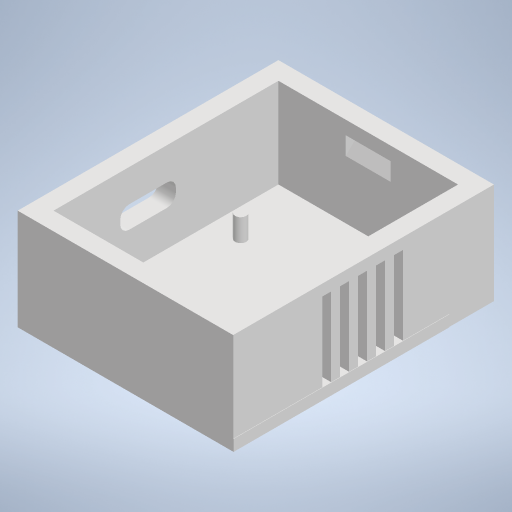
# Autodesk Inventor part: Unterseite
Saved by Autodesk Inventor 2024 (Build 280153000, 153)
## iProperties
Created: 2025-04-30
Part Number: Unterseite
Material: Generisch
Document SubType Name: Modeling
Designer: tobia
Density: 1 g/cm^3
Appearance: Vorgabe
Author: tobia
Autodesk Inventor part; units mm, degrees
ref_plane "YZ Plane" through (0, 0, 0) normal (1, 0, 0) x (0, 1, 0)
ref_plane "XZ Plane" through (0, 0, 0) normal (0, 1, 0) x (-1, 0, 0)
ref_plane "XY Plane" through (0, 0, 0) normal (0, 0, 1) x (1, 0, 0)
sketch "Skizze2" plane through (0, 0, 0) normal (0, 0, 1) x (1, 0, 0)
  line L0 (-24.05, 24.05) -> (24.05, 24.05)
  line L1 (24.05, 24.05) -> (24.05, -24.05)
  line L2 (24.05, -24.05) -> (-24.05, -24.05)
  line L3 (-24.05, -24.05) -> (-24.05, 24.05)
  line L4 (-24.05, 24.05) -> (24.05, -24.05) construction
  line L5 (24.05, 24.05) -> (-24.05, -24.05) construction
  line L6 (24.05, 24.05) -> (20.05, 24.05)
  line L7 (20.05, 24.05) -> (20.05, -24.05)
  line L8 (20.05, -24.05) -> (24.05, -24.05)
  line L9 (24.05, -24.05) -> (24.05, 24.05)
  line L10 (20.05, 24.05) -> (-24.05, 24.05)
  line L11 (-24.05, 24.05) -> (-24.05, 20.05)
  line L12 (-24.05, 20.05) -> (20.05, 20.05)
  line L13 (20.05, 20.05) -> (20.05, 24.05)
  line L14 (-24.05, 20.05) -> (-20.05, 20.05)
  line L15 (-20.05, 20.05) -> (-20.05, -24.05)
  line L16 (-20.05, -24.05) -> (-24.05, -24.05)
  line L17 (-24.05, -24.05) -> (-24.05, 20.05)
  line L18 (-20.05, -24.05) -> (20.05, -24.05)
  line L19 (20.05, -24.05) -> (20.05, -20.05)
  line L20 (20.05, -20.05) -> (-20.05, -20.05)
  line L21 (-20.05, -20.05) -> (-20.05, -24.05)
  point P0 (0, 0)
  dimension "d6" = 48.1
  dimension "d7" = 48.1
  dimension "d8" = 4
  dimension "d9" = 4
  dimension "d10" = 4
  dimension "d11" = 4
  constraints: 44 end point, 10 parallel, 5 horizontal, 5 perpendicular, 4 point on line, 2 midpoint
  measures "d6" distance of L1.end L2.end
  measures "d7" distance of L0.end L1.end
  measures "d8" distance of L8.end L7.end
  measures "d9" distance of L11.end L10.end
  measures "d10" distance of L15.end L16.end
  measures "d11" distance of L19.end L18.end
extrude "Extrusion1" add sketch "Skizze2" against normal blind 2.5
sketch "Skizze3" plane through (0, 0, 0) normal (0, 0, 1) x (1, 0, 0)
  line L0 (-24.05, -24.05) -> (-24.05, 24.05) projected
  line L1 (-24.05, 24.05) -> (-20.05, 24.05)
  line L2 (-20.05, 24.05) -> (-20.05, -24.05)
  line L3 (-20.05, -24.05) -> (-24.05, -24.05)
  line L4 (-24.05, -24.05) -> (-24.05, 24.05)
  line L5 (24.05, 24.05) -> (24.05, -24.05) projected
  line L6 (24.05, 24.05) -> (20.05, 24.05)
  line L7 (20.05, 24.05) -> (20.05, -24.05)
  line L8 (20.05, -24.05) -> (24.05, -24.05)
  line L9 (24.05, -24.05) -> (24.05, 24.05)
  line L10 (20.05, -24.05) -> (-20.05, -24.05)
  line L11 (-20.05, -24.05) -> (-20.05, -20.05)
  line L12 (-20.05, -20.05) -> (20.05, -20.05)
  line L13 (20.05, -20.05) -> (20.05, -24.05)
  line L14 (-20.05, 24.05) -> (20.05, 24.05)
  line L15 (20.05, 24.05) -> (20.05, 20.05)
  line L16 (20.05, 20.05) -> (-20.05, 20.05)
  line L17 (-20.05, 20.05) -> (-20.05, 24.05)
  circle A0 centre (1.0405, -13.9467) radius 1.25
  circle A1 centre (14.1846, 15.3896) radius 1.25
  circle A2 centre (-13.8014, 15.3896) radius 1.25
  point P0 (0, 0)
  dimension "d14" = 4
  dimension "d15" = 4
  dimension "d16" = 4
  dimension "d17" = 4
  dimension "d18" = 2.5
  dimension "d19" = 2.5
  dimension "d20" = 2.5
  constraints: 32 end point, 8 parallel, 4 horizontal, 4 perpendicular, 3 centre point, 3 point on line
  measures "d14" distance of L2.end L3.end
  measures "d15" distance of L8.end L7.end
  measures "d16" distance of L10.end L11.end
  measures "d17" distance of L14.end L15.end
  measures "d18" diameter of A0
  measures "d19" diameter of A1
  measures "d20" diameter of A2
extrude "Extrusion2" add sketch "Skizze3" along normal blind 2.5 contours A0 | A1 | A2
sketch "Skizze4" plane through (-13.8014, 15.3896, 2.5) normal (0, 0, 1) x (1, 0, 0)
  circle A0 centre (27.986, 0) radius 1.25 projected
  circle A1 centre (27.986, 0) radius 1.25
  circle A2 centre (0, 0) radius 1.25 projected
  circle A3 centre (0, 0) radius 1.25
  circle A4 centre (14.8419, -29.3364) radius 1.25 projected
  circle A5 centre (14.8419, -29.3364) radius 1.25
  point P0 (13.8014, -15.3896)
  constraints: 3 centre point, 3 coincident
extrude "Extrusion3" add sketch "Skizze4" along normal blind 2.5
sketch "Skizze5" plane through (-24.05, 24.05, 0) normal (0, 1, 0) x (1, 0, 0)
  line L0 (48.1, 2.5) -> (0, 2.5) projected
  line L1 (48.0134, 0) -> (0, 0)
  line L2 (0, 0) -> (0, 2.5)
  line L3 (0, 2.5) -> (48.0134, 2.5)
  line L4 (48.0134, 2.5) -> (48.0134, 0)
  point P0 (24.05, 0)
  constraints: 8 end point, 2 parallel, 1 horizontal, 1 perpendicular
extrude "Extrusion4" add sketch "Skizze5" along normal blind 10
sketch "Skizze6" plane through (0, 0, 0) normal (0, 0, 1) x (1, 0, 0)
  line L0 (24.05, -24.05) -> (-24.05, -24.05) projected
  line L1 (23.9634, 34.05) -> (-24.05, 34.05) projected
  line L2 (-24.05, -24.05) -> (-20.05, -24.05)
  line L3 (-20.05, -24.05) -> (-20.05, 34.05)
  line L4 (-20.05, 34.05) -> (-24.05, 34.05)
  line L5 (-24.05, 34.05) -> (-24.05, -24.05)
  line L6 (23.9634, 24.05) -> (23.9634, 34.05) projected
  line L7 (-20.05, 34.05) -> (23.9634, 34.05)
  line L8 (23.9634, 34.05) -> (23.9634, 30.05)
  line L9 (23.9634, 30.05) -> (-20.05, 30.05)
  line L10 (-20.05, 30.05) -> (-20.05, 34.05)
  line L11 (23.9634, 30.05) -> (19.9634, 30.05)
  line L12 (19.9634, 30.05) -> (19.9634, -24.05)
  line L13 (19.9634, -24.05) -> (23.9634, -24.05)
  line L14 (23.9634, -24.05) -> (23.9634, 30.05)
  line L15 (19.9634, -24.05) -> (-20.05, -24.05)
  line L16 (-20.05, -24.05) -> (-20.05, -20.05)
  line L17 (-20.05, -20.05) -> (19.9634, -20.05)
  line L18 (19.9634, -20.05) -> (19.9634, -24.05)
  point P0 (0, 0)
  point P1 (-20.05, 30.05)
  dimension "d27" = 4
  dimension "d28" = 4
  dimension "d29" = 4
  dimension "d30" = 4
  constraints: 32 end point, 8 parallel, 4 horizontal, 4 perpendicular, 4 point on line
  measures "d27" distance of L4.end L3.end
  measures "d28" distance of L7.end L8.end
  measures "d29" distance of L13.end L12.end
  measures "d30" distance of L15.end L16.end
extrude "Extrusion5" add sketch "Skizze6" along normal blind 20 contours L0 L12 L9 L6 L14 | L0 L3 L17 L12 | L0 L5 L1 L3 | L9 L3 L1 L6
sketch "Skizze8" plane through (-20.05, -20.05, 0) normal (1, 0, 0) x (0, 0, -1)
  line L0 (-12.8089, 14.8489) -> (-7.8985, 14.8489)
  line L1 (-7.8985, 14.8489) -> (-7.8985, 27.2593)
  line L2 (-7.8985, 27.2593) -> (-12.8089, 27.2593)
  line L3 (-12.8089, 27.2593) -> (-12.8089, 14.8489)
  line L4 (-12.8089, 14.8489) -> (-7.8985, 27.2593) construction
  line L5 (-7.8985, 14.8489) -> (-12.8089, 27.2593) construction
  point P0 (0, 20.05)
  point P1 (-10.3537, 21.0541)
  constraints: 12 end point, 2 midpoint, 2 parallel, 1 horizontal, 1 perpendicular
extrude "Extrusion6" cut sketch "Skizze8" against normal blind 20
fillet "Rundung1" radius 2 4 edges at (-22.05, -5.2011, 12.8089) (-22.05, -5.2011, 7.8985) (-22.05, 7.2093, 12.8089) (-22.05, 7.2093, 7.8985)
sketch "Skizze9" plane through (23.9634, 24.05, 0) normal (1, 0, 0) x (0, 0, -1)
  line L0 (2.5, 10) -> (-20, 10) projected
  line L1 (-20, -48.1) -> (-17.5, -48.1)
  line L2 (-17.5, -48.1) -> (-17.5, 10)
  line L3 (-17.5, 10) -> (-20, 10)
  line L4 (-20, 10) -> (-20, -48.1)
  line L5 (0, -48.1) -> (0, 0) projected
  line L6 (0, -12.2697) -> (-17.5, -12.2697)
  line L7 (-17.5, -12.2697) -> (0, -12.2697)
  line L8 (0, -12.2697) -> (0, -14.2697)
  line L9 (0, -14.2697) -> (-17.5, -14.2697)
  line L10 (-17.5, -14.2697) -> (-17.5, -12.2697)
  line L11 (0, -14.2697) -> (-17.5, -14.2697)
  line L12 (-17.5, -14.2697) -> (-17.5, -16.2697)
  line L13 (-17.5, -16.2697) -> (0, -16.2697)
  line L14 (0, -16.2697) -> (0, -14.2697)
  line L15 (-17.5, -16.2697) -> (0, -16.2697)
  line L16 (0, -16.2697) -> (0, -18.2697)
  line L17 (0, -18.2697) -> (-17.5, -18.2697)
  line L18 (-17.5, -18.2697) -> (-17.5, -16.2697)
  line L19 (0, -18.2697) -> (-17.5, -18.2697)
  line L20 (-17.5, -18.2697) -> (-17.5, -20.2697)
  line L21 (-17.5, -20.2697) -> (0, -20.2697)
  line L22 (0, -20.2697) -> (0, -18.2697)
  line L23 (-17.5, -20.2697) -> (0, -20.2697)
  line L24 (0, -20.2697) -> (0, -22.2697)
  line L25 (0, -22.2697) -> (-17.5, -22.2697)
  line L26 (-17.5, -22.2697) -> (-17.5, -20.2697)
  line L27 (0, -22.2697) -> (-17.5, -22.2697)
  line L28 (-17.5, -22.2697) -> (-17.5, -24.2697)
  line L29 (-17.5, -24.2697) -> (0, -24.2697)
  line L30 (0, -24.2697) -> (0, -22.2697)
  line L31 (-17.5, -24.2697) -> (0, -24.2697)
  line L32 (0, -24.2697) -> (0, -26.2697)
  line L33 (0, -26.2697) -> (-17.5, -26.2697)
  line L34 (-17.5, -26.2697) -> (-17.5, -24.2697)
  line L35 (0, -26.2697) -> (-17.5, -26.2697)
  line L36 (-17.5, -26.2697) -> (-17.5, -28.2697)
  line L37 (-17.5, -28.2697) -> (0, -28.2697)
  line L38 (0, -28.2697) -> (0, -26.2697)
  line L39 (-17.5, -12.2697) -> (0, -12.2697)
  line L40 (0, -12.2697) -> (0, -10.2697)
  line L41 (0, -10.2697) -> (-17.5, -10.2697)
  line L42 (-17.5, -10.2697) -> (-17.5, -12.2697)
  point P0 (0, -24.05)
  dimension "d36" = 2.5
  dimension "d38" = 2
  dimension "d39" = 2
  dimension "d40" = 2
  dimension "d41" = 2
  dimension "d42" = 2
  dimension "d43" = 2
  dimension "d44" = 2
  dimension "d45" = 2
  dimension "d46" = 2
  constraints: 82 end point, 20 parallel, 10 horizontal, 10 perpendicular, 5 point on line, 7 other
  measures "d36" distance of L3.end L2.end
  measures "d38" distance of L7.end L8.end
  measures "d39" distance of L12.end L11.end
  measures "d40" distance of L15.end L16.end
  measures "d41" distance of L20.end L19.end
  measures "d42" distance of L23.end L24.end
  measures "d43" distance of L28.end L27.end
  measures "d44" distance of L31.end L32.end
  measures "d45" distance of L36.end L35.end
  measures "d46" distance of L40.end L39.end
extrude "Extrusion7" cut sketch "Skizze9" against normal blind 20 contours L41 L5 L6 L2 | L9 L5 L13 L2 | L2 L33 L5 L37 | L17 L5 L21 L2 | L2 L25 L5 L29
sketch "Skizze10" plane through (-20.05, -20.05, 0) normal (0, 1, 0) x (1, 0, 0)
  line L0 (40.0134, 0) -> (40.0134, -20) projected
  line L1 (40.0134, -20) -> (20.0134, -20)
  line L2 (0, 0) -> (0, -20) projected
  line L3 (20.0134, -20) -> (20.0134, -15)
  line L4 (25.0134, -17) -> (15.0134, -17)
  line L5 (15.0134, -17) -> (15.0134, -13)
  line L6 (15.0134, -13) -> (25.0134, -13)
  line L7 (25.0134, -13) -> (25.0134, -17)
  line L8 (25.0134, -17) -> (15.0134, -13) construction
  line L9 (15.0134, -17) -> (25.0134, -13) construction
  line L10 (25.0134, -17) -> (25.0134, -15)
  line L11 (25.0134, -15) -> (15.0134, -15)
  point P0 (20.05, 0)
  dimension "d49" = 20
  dimension "d50" = 5
  dimension "d51" = 10
  dimension "d52" = 4
  dimension "d53" = 2
  constraints: 20 end point, 4 midpoint, 2 parallel, 2 perpendicular, 1 horizontal, 1 vertical
  measures "d49" distance of L0.end L1.end
  measures "d50" distance of L1.end L3.end
  measures "d51" distance of L5.end L6.end
  measures "d52" distance of L4.end L5.end
  measures "d53" distance of L4.start L10.end
extrude "Extrusion8" cut sketch "Skizze10" against normal blind 2
chamfer "Fasen1" distance 2 angle 45 2 edges at (-0.0366, -22.05, 17) (-0.0366, -22.05, 13)
sketch "Skizze12" plane through (-20.05, 30.05, 0) normal (0, -1, 0) x (1, 0, 0)
  line L0 (40.0134, 0) -> (40.0134, 20) projected
  line L1 (40.0134, 20) -> (20.0134, 20)
  line L2 (0, 20) -> (40.0134, 20) projected
  line L3 (20.0134, 20) -> (20.0134, 15)
  line L4 (15.0134, 17) -> (25.0134, 17)
  line L5 (25.0134, 17) -> (25.0134, 13)
  line L6 (25.0134, 13) -> (15.0134, 13)
  line L7 (15.0134, 13) -> (15.0134, 17)
  line L8 (15.0134, 17) -> (25.0134, 13) construction
  line L9 (25.0134, 17) -> (15.0134, 13) construction
  line L10 (20.0134, 15) -> (15.0134, 15)
  line L11 (20.0134, 15) -> (25.0134, 15)
  point P0 (20.05, 0)
  dimension "d59" = 20
  dimension "d60" = 5
  dimension "d61" = 10
  dimension "d62" = 4
  constraints: 20 end point, 4 midpoint, 2 parallel, 2 perpendicular, 1 horizontal, 1 point on line
  measures "d59" distance of L0.end L1.end
  measures "d60" distance of L1.end L3.end
  measures "d61" distance of L5.end L6.end
  measures "d62" distance of L4.end L5.end
extrude "Extrusion9" cut sketch "Skizze12" against normal blind 2
chamfer "Fasen2" distance 2 angle 45 2 edges at (-0.0366, 32.05, 13) (-0.0366, 32.05, 17)
